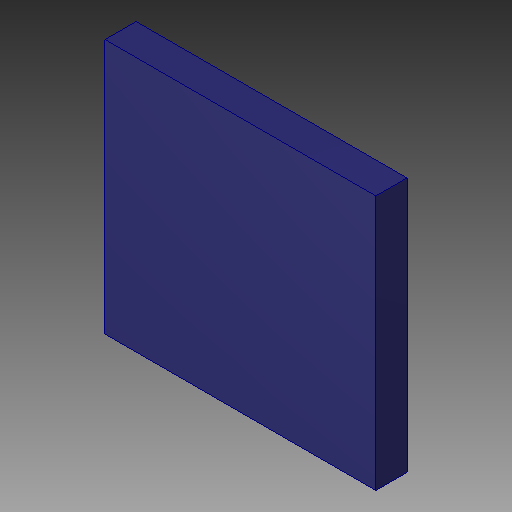
# Autodesk Inventor part: GBA-LINK
Saved by Autodesk Inventor 2017 (Build 210142000, 142)
## iProperties
Created: 2022-08-30
Part Number: GBA-LINK
Material: Generic
Document SubType Name: Modeling
Designer: Collin
Density: 1 g/cm^3
Appearance: GBA-LINK, GBA-LINK
Author: Collin
Autodesk Inventor part; units mm, degrees
ref_plane "YZ Plane" through (0, 0, 0) normal (1, 0, 0) x (0, 1, 0)
ref_plane "XZ Plane" through (0, 0, 0) normal (0, 1, 0) x (-1, 0, 0)
ref_plane "XY Plane" through (0, 0, 0) normal (0, 0, 1) x (1, 0, 0)
sketch "GBA-LINK, GBA-LINK_1" plane through (0, 0, 0) normal (0, 0, 1) x (1, 0, 0)
  line L0 (-4.3815, 0.127) -> (4.318, 0.127)
  line L1 (4.318, 0.127) -> (4.318, -8.0645)
  line L2 (4.318, -8.0645) -> (-4.3815, -8.0645)
  line L3 (-4.3815, -8.0645) -> (-4.3815, 0.127)
  constraints: 8 end point
extrude "Extrusion1" add sketch "GBA-LINK, GBA-LINK_1" along normal blind 1
body "Solid1"
